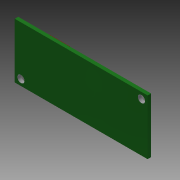
# Autodesk Inventor part: modemode
Saved by Autodesk Inventor 2015 (Build 190159000, 159)
## iProperties
Created: 2015-02-04
Part Number: modemode
Material: Generic
Document SubType Name: Modeling
Designer: Rafi Kurnia Putra
Density: 1 g/cm^3
Appearance: Default
Mass: 3.92593 g
Surface Area: 48.0387 cm^2
Volume: 3.92593 cm^3
Author: Rafi Kurnia Putra
Autodesk Inventor part; units mm, degrees
ref_plane "YZ Plane" through (0, 0, 0) normal (1, 0, 0) x (0, 1, 0)
ref_plane "XZ Plane" through (0, 0, 0) normal (0, 1, 0) x (-1, 0, 0)
ref_plane "XY Plane" through (0, 0, 0) normal (0, 0, 1) x (1, 0, 0)
sketch "Sketch1" plane through (0, 0, 0) normal (0, 1, 0) x (-1, 0, 0)
  line L0 (32.512, 13.5) -> (-32.512, 13.5)
  line L1 (-32.512, 13.5) -> (-32.512, -13.5)
  line L2 (-32.512, -13.5) -> (32.512, -13.5)
  line L3 (32.512, -13.5) -> (32.512, 13.5)
  line L4 (32.512, 13.5) -> (-32.512, -13.5) construction
  line L5 (-32.512, 13.5) -> (32.512, -13.5) construction
  circle A0 centre (29.512, -10.5) radius 1.75
  circle A1 centre (-29.512, 10.5) radius 1.75
  line L6 (24.13, 6.6847) -> (14.17, 6.6847)
  line L7 (14.17, 6.6847) -> (14.17, -4.9753)
  line L8 (14.17, -4.9753) -> (24.13, -4.9753)
  line L9 (24.13, -4.9753) -> (24.13, 6.6847)
  line L10 (24.13, 6.6847) -> (14.17, -4.9753) construction
  line L11 (14.17, 6.6847) -> (24.13, -4.9753) construction
  circle A2 centre (25.575, -9.23) radius 0.5
  point P0 (0, 0)
  point P1 (19.15, 0.8547)
  dimension "d0" = 65.024
  dimension "d1" = 27
  dimension "d2" = 3.5
  dimension "d3" = 3.5
  dimension "d4" = 3
  dimension "d5" = 3
  dimension "d6" = 3
  dimension "d7" = 3
  dimension "d8" = 9.96
  dimension "d9" = 11.66
  dimension "d10" = 1
  dimension "d11" = 1.27
  dimension "d12" = 3.937
  constraints: 24 end point, 4 midpoint, 4 parallel, 3 centre point, 2 horizontal, 2 perpendicular
  measures "d0" distance of L2.end L1.end
  measures "d1" distance of L1.end L0.end
  measures "d2" diameter of A0
  measures "d3" diameter of A1
  measures "d4" distance from line of A0.centre L3
  measures "d5" distance from line of A0.centre L2
  measures "d6" distance from line of L1 A1.centre
  measures "d7" distance from line of A1.centre L0
  measures "d8" distance of L8.end L7.end
  measures "d9" distance of L7.end L6.end
  measures "d10" diameter of A2
  measures "d11" vertical distance of A2.centre A0.centre
  measures "d12" horizontal distance of A2.centre A0.centre
extrude "Extrusion1" add sketch "Sketch1" along normal blind 1.7
extrude "Extrusion2" add sketch "Sketch1" along normal blind 8.62 contours L9 L8 L7 L6
sketch "Sketch2" plane through (32.512, 0, 13.5) normal (1, 0, 0) x (0, 0, -1)
  line L0 (0, 0) -> (27, 0) projected
  line L1 (24.3183, 0) -> (24.3183, 6.15)
  line L2 (24.3183, 0) -> (30.4683, 0) construction
  line L3 (24.3183, 6.15) -> (32.1883, 6.15)
  point P0 (13.5, 0)
  dimension "d17" = 6.15
  dimension "d18" = 90
  dimension "d19" = 7.87
  dimension "d20" = 90
  constraints: 6 end point, 2 perpendicular, 1 horizontal, 1 point on line, 1 vertical
  measures "d17" distance of L1.start L1.end
  measures "d18" angle of L2 L1
  measures "d19" distance of L1.end L3.end
  measures "d20" angle of L1 L3
sweep "Sweep1" add profiles "Sketch1" path "Sketch2" path curves L1 L3 contours A2
pattern_linear "Rectangular Pattern1" count 18 spacing 2.54 along (1, 0, 0) of "Sweep1" skipped copies 4 10 11 12
sketch "Sketch3" plane through (0, 1.7, 0) normal (0, 1, 0) x (1, 0, 0)
  line L0 (-11.9382, 1.4781) -> (29.8264, 1.4781) construction
  line L1 (29.8264, 1.4781) -> (29.8264, -2.1694) construction
  line L2 (29.8264, -2.1694) -> (-11.9382, -2.1694) construction
  line L3 (-11.9382, -2.1694) -> (-11.9382, 1.4781) construction
  point P0 (0, 0)
  constraints: 2 other
body "Solid1"
